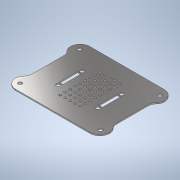
# Autodesk Inventor part: spacer
Saved by Autodesk Inventor 2022 (Build 260153000, 153)
## iProperties
Created: 2021-07-16
Part Number: spacer
Material: Stainless Steel
Document SubType Name: Modeling
Designer: Caleb
Density: 8 g/cm^3
Appearance: Semi-Polished
Author: Caleb
Autodesk Inventor part; units mm, degrees
ref_plane "YZ Plane" through (0, 0, 0) normal (1, 0, 0) x (0, 1, 0)
ref_plane "XZ Plane" through (0, 0, 0) normal (0, 1, 0) x (-1, 0, 0)
ref_plane "XY Plane" through (0, 0, 0) normal (0, 0, 1) x (1, 0, 0)
sketch "Sketch1" plane through (0, 0, 0) normal (0, 1, 0) x (-1, 0, 0)
  line L0 (-23.8125, 23.8125) -> (23.8125, 23.8125)
  line L1 (30.1625, 17.4625) -> (30.1625, -17.4625)
  line L2 (23.8125, -23.8125) -> (-23.8125, -23.8125)
  line L3 (-30.1625, -17.4625) -> (-30.1625, 17.4625)
  line L4 (-30.1625, 23.8125) -> (30.1625, -23.8125) construction
  line L5 (30.1625, 23.8125) -> (-30.1625, -23.8125) construction
  arc A0 (30.1625, 17.4625) -> (23.8125, 23.8125) centre (23.8125, 17.4625) ccw
  arc A1 (23.8125, -23.8125) -> (30.1625, -17.4625) centre (23.8125, -17.4625) ccw
  arc A2 (-30.1625, -17.4625) -> (-23.8125, -23.8125) centre (-23.8125, -17.4625) ccw
  arc A3 (-23.8125, 23.8125) -> (-30.1625, 17.4625) centre (-23.8125, 17.4625) ccw
  point P0 (0, 0)
  dimension "d0" = 47.625
  dimension "d1" = 60.325
  dimension "d2" = 6.35
  constraints: 12 end point, 8 point on circle, 8 point on line, 8 tangent, 4 centre point, 3 equal radius, 2 midpoint, 2 parallel, 1 horizontal, 1 perpendicular
  measures "d0" distance of L5.start L4.end
  measures "d1" distance of L4.end L5.end
  measures "d2" radius of A0
extrude "Extrusion1" add sketch "Sketch1" along normal blind 0.743
sketch "Sketch2" plane through (0, 0.743, 0) normal (0, 1, 0) x (1, 0, 0)
  point P0 (0, 0)
  point P1 (-25.8, 19.1)
  point P2 (25.8, 19.1)
  point P3 (-25.8, -19.1)
  point P4 (25.8, -19.1)
  dimension "d5" = 25.8
  dimension "d6" = 19.1
  dimension "d7" = 19.1
  dimension "d8" = 25.8
  constraints: 2 horizontal alignment, 2 vertical alignment
  measures "d5" horizontal distance of point (0, 0) point (-25.8, 19.1)
  measures "d6" vertical distance of point (-25.8, 19.1) point (0, 0)
  measures "d7" vertical distance of point (0, 0) point (25.8, -19.1)
  measures "d8" horizontal distance of point (0, 0) point (25.8, -19.1)
hole "Hole1" at (-25.8, 0.743, -19.1) at (25.8, 0.743, -19.1) at (-25.8, 0.743, 19.1) at (25.8, 0.743, 19.1) direction (0, -1, 0) diameter 2.5 end through all
sketch "Sketch3" plane through (0, 0.743, 0) normal (0, 1, 0) x (1, 0, 0)
  line L0 (-11.43, -5.969) -> (-13.97, -5.969)
  line L1 (-13.97, -5.969) -> (-13.97, 5.969)
  line L2 (-13.97, 5.969) -> (-11.43, 5.969)
  line L3 (-11.43, 5.969) -> (-11.43, -5.969)
  line L4 (-11.43, -5.969) -> (-13.97, 5.969) construction
  line L5 (-13.97, -5.969) -> (-11.43, 5.969) construction
  line L6 (13.97, -5.969) -> (11.43, -5.969)
  line L7 (11.43, -5.969) -> (11.43, 5.969)
  line L8 (11.43, 5.969) -> (13.97, 5.969)
  line L9 (13.97, 5.969) -> (13.97, -5.969)
  line L10 (13.97, -5.969) -> (11.43, 5.969) construction
  line L11 (11.43, -5.969) -> (13.97, 5.969) construction
  point P0 (0, 0)
  point P1 (-12.7, 0)
  point P2 (12.7, 0)
  point P3 (-12.7, 0)
  point P4 (12.7, 0)
  point P5 (-12.7, 0)
  dimension "d18" = 11.938
  dimension "d21" = 2.54
  dimension "d22" = 11.43
  dimension "d23" = 11.43
  constraints: 24 end point, 7 midpoint, 4 parallel, 2 equal length, 2 horizontal, 2 horizontal alignment, 2 perpendicular, 1 coincident
  measures "d18" distance of L0.end L1.end
  measures "d21" distance of L0.start L0.end
  measures "d22" horizontal distance of point (0, 0) L2.end
  measures "d23" horizontal distance of L7.end point (0, 0)
extrude "Extrusion2" cut sketch "Sketch3" against normal through all
sketch "Sketch4" plane through (0, 0.743, 0) normal (0, 1, 0) x (1, 0, 0)
  line L0 (0, -6.7565) -> (0, 0)
  line L1 (5.4145, 0) -> (0, 0)
  point P0 (-6.35, -12.7)
  point P1 (-6.35, -9.525)
  point P2 (-6.35, -6.35)
  point P3 (-6.35, -3.175)
  point P4 (-6.35, 0)
  point P5 (-6.35, 3.175)
  point P6 (-6.35, 6.35)
  point P7 (-6.35, 9.525)
  point P8 (-6.35, 12.7)
  point P9 (-3.175, -12.7)
  point P10 (-3.175, -9.525)
  point P11 (-3.175, -6.35)
  point P12 (-3.175, -3.175)
  point P13 (-3.175, 0)
  point P14 (-3.175, 3.175)
  point P15 (-3.175, 6.35)
  point P16 (-3.175, 9.525)
  point P17 (-3.175, 12.7)
  point P18 (0, -12.7)
  point P19 (0, -9.525)
  point P20 (0, -6.35)
  point P21 (0, -3.175)
  point P22 (0, 3.175)
  point P23 (0, 6.35)
  point P24 (0, 9.525)
  point P25 (0, 12.7)
  point P26 (3.175, -12.7)
  point P27 (3.175, -9.525)
  point P28 (3.175, -6.35)
  point P29 (3.175, -3.175)
  point P30 (3.175, 0)
  point P31 (3.175, 3.175)
  point P32 (3.175, 6.35)
  point P33 (3.175, 9.525)
  point P34 (3.175, 12.7)
  point P35 (6.35, -12.7)
  point P36 (6.35, -9.525)
  point P37 (6.35, -6.35)
  point P38 (6.35, -3.175)
  point P39 (6.35, 0)
  point P40 (6.35, 3.175)
  point P41 (6.35, 6.35)
  point P42 (6.35, 9.525)
  point P43 (6.35, 12.7)
  dimension "d24" = 12.7
  dimension "d25" = 6.35
  dimension "d28" = 3.175
  dimension "d31" = 3.175
  constraints: 4 end point, 2 horizontal, 2 vertical, 44 other
  measures "d24" vertical distance of point (-6.35, -12.7) L0.end
  measures "d25" horizontal distance of L0.end point (-6.35, -12.7)
  measures "d28" distance of point (-6.35, -12.7) point (-6.35, -9.525)
  measures "d31" distance of point (-6.35, -12.7) point (-3.175, -12.7)
hole "Hole2" at (-6.35, 0.743, 12.7) at (-6.35, 0.743, 9.525) at (-6.35, 0.743, 6.35) at (-6.35, 0.743, 3.175) at (-6.35, 0.743, 0) at (-6.35, 0.743, -3.175) at (-6.35, 0.743, -6.35) at (-6.35, 0.743, -9.525) at (-6.35, 0.743, -12.7) at (-3.175, 0.743, 12.7) at (-3.175, 0.743, 9.525) at (-3.175, 0.743, 6.35) at (-3.175, 0.743, 3.175) at (-3.175, 0.743, 0) at (-3.175, 0.743, -3.175) at (-3.175, 0.743, -6.35) at (-3.175, 0.743, -9.525) at (-3.175, 0.743, -12.7) at (0, 0.743, 12.7) at (0, 0.743, 9.525) at (0, 0.743, 6.35) at (0, 0.743, 3.175) at (0, 0.743, 0) at (0, 0.743, -3.175) at (0, 0.743, -6.35) at (0, 0.743, -9.525) at (0, 0.743, -12.7) at (3.175, 0.743, 12.7) at (3.175, 0.743, 9.525) at (3.175, 0.743, 6.35) at (3.175, 0.743, 3.175) at (3.175, 0.743, 0) at (3.175, 0.743, -3.175) at (3.175, 0.743, -6.35) at (3.175, 0.743, -9.525) at (3.175, 0.743, -12.7) at (6.35, 0.743, 12.7) at (6.35, 0.743, 9.525) at (6.35, 0.743, 6.35) at (6.35, 0.743, 3.175) at (6.35, 0.743, 0) at (6.35, 0.743, -3.175) at (6.35, 0.743, -6.35) at (6.35, 0.743, -9.525) at (6.35, 0.743, -12.7) direction (0, -1, 0) diameter 1.5875 end through all
sketch "Sketch5" plane through (0, 0.743, 0) normal (0, 1, 0) x (1, 0, 0)
  line L0 (-30.1625, 17.4625) -> (-30.1625, -17.4625) projected
  line L1 (30.1625, -17.4625) -> (30.1625, 17.4625) projected
  arc A0 (-23.8125, 23.8125) -> (-30.1625, 17.4625) centre (-23.8125, 17.4625) ccw projected
  arc A1 (-30.1625, -17.4625) -> (-23.8125, -23.8125) centre (-23.8125, -17.4625) ccw projected
  arc A2 (-28.6746, -13.8704) -> (-30.1625, -17.4625) centre (-25.0825, -17.4625) ccw
  line L2 (-30.1625, -17.4625) -> (-25.0825, -17.4625) construction
  line L3 (-28.6746, -13.8704) -> (-25.0825, -17.4625) construction
  arc A3 (-28.6746, -13.8704) -> (-27.1867, -10.2783) centre (-32.2667, -10.2783) ccw
  line L4 (-28.6746, -13.8704) -> (-32.2667, -10.2783) construction
  line L5 (-27.1867, -10.2783) -> (-32.2667, -10.2783) construction
  arc A4 (-30.1625, 17.4625) -> (-28.6746, 13.8704) centre (-25.0825, 17.4625) ccw
  line L6 (-30.1625, 17.4625) -> (-25.0825, 17.4625) construction
  line L7 (-28.6746, 13.8704) -> (-25.0825, 17.4625) construction
  arc A5 (-27.1867, 10.2783) -> (-28.6746, 13.8704) centre (-32.2667, 10.2783) ccw
  line L8 (-28.6746, 13.8704) -> (-32.2667, 10.2783) construction
  line L9 (-27.1867, 10.2783) -> (-32.2667, 10.2783) construction
  line L10 (-27.1867, 10.2783) -> (-27.1867, -10.2783)
  arc A6 (30.1625, 17.4625) -> (23.8125, 23.8125) centre (23.8125, 17.4625) ccw projected
  arc A7 (23.8125, -23.8125) -> (30.1625, -17.4625) centre (23.8125, -17.4625) ccw projected
  arc A8 (28.6746, 13.8704) -> (30.1625, 17.4625) centre (25.0825, 17.4625) ccw
  line L11 (30.1625, 17.4625) -> (25.0825, 17.4625) construction
  line L12 (28.6746, 13.8704) -> (25.0825, 17.4625) construction
  arc A9 (28.6746, 13.8704) -> (27.1867, 10.2783) centre (32.2667, 10.2783) ccw
  line L13 (28.6746, 13.8704) -> (32.2667, 10.2783) construction
  line L14 (27.1867, 10.2783) -> (32.2667, 10.2783) construction
  arc A10 (30.1625, -17.4625) -> (28.6746, -13.8704) centre (25.0825, -17.4625) ccw
  line L15 (30.1625, -17.4625) -> (25.0825, -17.4625) construction
  line L16 (28.6746, -13.8704) -> (25.0825, -17.4625) construction
  arc A11 (27.1867, -10.2783) -> (28.6746, -13.8704) centre (32.2667, -10.2783) ccw
  line L17 (28.6746, -13.8704) -> (32.2667, -10.2783) construction
  line L18 (27.1867, -10.2783) -> (32.2667, -10.2783) construction
  line L19 (27.1867, -10.2783) -> (27.1867, 10.2783)
  point P0 (0, 0)
  dimension "d41" = 5.08
  dimension "d42" = 45
  dimension "d43" = 5.08
  dimension "d44" = 45
  dimension "d45" = 5.08
  dimension "d46" = 45
  dimension "d47" = 5.08
  dimension "d48" = 45
  dimension "d51" = 5.08
  dimension "d52" = 45
  dimension "d53" = 5.08
  dimension "d54" = 45
  dimension "d57" = 5.08
  dimension "d58" = 45
  dimension "d59" = 5.08
  dimension "d60" = 45
  constraints: 36 end point, 16 point on circle, 8 centre point, 8 tangent
  measures "d41" radius of A2
  measures "d42" angle of L3 L2
  measures "d43" radius of A3
  measures "d44" angle of L4 L5
  measures "d45" radius of A4
  measures "d46" angle of L6 L7
  measures "d47" radius of A5
  measures "d48" angle of L9 L8
  measures "d51" radius of A8
  measures "d52" angle of L12 L11
  measures "d53" radius of A9
  measures "d54" angle of L13 L14
  measures "d57" radius of A10
  measures "d58" angle of L15 L16
  measures "d59" radius of A11
  measures "d60" angle of L18 L17
extrude "Extrusion3" cut sketch "Sketch5" against normal through all
sketch "Sketch6" plane through (0, 0.743, 0) normal (0, 1, 0) x (1, 0, 0)
  point P0 (0, 0)
  point P1 (-12.7, 7.62)
  point P2 (-12.7, -7.62)
  point P3 (12.7, 7.62)
  point P4 (12.7, -7.62)
  dimension "d61" = 7.62
  dimension "d62" = 7.62
  dimension "d63" = 12.7
  dimension "d64" = 12.7
  constraints: 2 horizontal alignment, 2 vertical alignment
  measures "d61" vertical distance of point (0, 0) point (-12.7, 7.62)
  measures "d62" vertical distance of point (0, 0) point (-12.7, -7.62)
  measures "d63" horizontal distance of point (-12.7, 7.62) point (0, 0)
  measures "d64" horizontal distance of point (12.7, 7.62) point (0, 0)
hole "Hole3" at (-12.7, 0.743, -7.62) at (-12.7, 0.743, 7.62) at (12.7, 0.743, -7.62) at (12.7, 0.743, 7.62) direction (0, -1, 0) diameter 2.54 end through all
body "Solid1"
